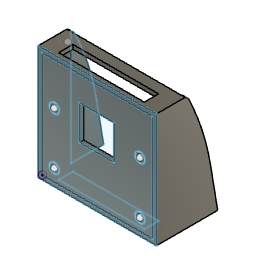
Drone_PiCameraCase v4 (Autodesk Fusion 360 design; units mm, degrees)
Autodesk Fusion 360 part; units mm, degrees
sketch "Sketch2" plane through (0, 0, 0) normal (0, 1, 0) x (1, 0, 0)
  circle A0 centre (2.9671, -2.9729) radius 1.2
  circle A1 centre (23.9671, -2.9729) radius 1.2
  circle A2 centre (23.9671, -15.7229) radius 1.2
  circle A3 centre (2.9671, -15.7229) radius 1.2
  line L0 (9.1497, -11.5214) -> (9.1497, -19.9214)
  line L1 (9.1497, -19.9214) -> (17.5497, -19.9214)
  line L2 (17.5497, -19.9214) -> (17.5497, -11.5214)
  line L3 (17.5497, -11.5214) -> (9.1497, -11.5214)
  line L4 (26.9671, 0.0271) -> (26.9671, -25.9729)
  line L5 (26.9671, -25.9729) -> (-0.0329, -25.9729)
  line L6 (-0.0329, -25.9729) -> (-0.0329, 0.0271)
  line L7 (-0.0329, 0.0271) -> (26.9671, 0.0271)
  line L8 (-1, -27) -> (28, -27)
  line L9 (28, -27) -> (28, 1)
  line L10 (28, 1) -> (-1, 1)
  line L11 (-1, 1) -> (-1, -27)
  dimension "d3" = 2.4
  dimension "d4" = 2.4
  dimension "d5" = 2.4
  dimension "d6" = 2.4
  dimension "d7" = 8.4
  dimension "d8" = 8.4
  constraint horizontal L8
  constraint vertical L9
  constraint horizontal L10
  constraint vertical L11
  measures "d3" diameter of A0
  measures "d4" diameter of A1
  measures "d5" diameter of A2
  measures "d6" diameter of A3
  measures "d7" distance of L0.start L0.end
  measures "d8" distance of L0.start L2.end
extrude "Extrude12" add sketch "Sketch2" along normal blind 1 contours L4 L5 L6 L7 makes body 1
extrude "Extrude11" add sketch "Sketch2" along normal blind 7 separate body contours L8 L9 L10 L11 makes body 2
extrude "Extrude13" add sketch "Sketch2" along normal blind 5 contours A0 | A1 | A2 | A3 bodies 1
sketch "Sketch5" plane through (0, 0, 0) normal (0, 0, 1) x (1, 0, 0)
  line L0 (3, 4.5) -> (24, 4.5)
  line L1 (24, 4.5) -> (24, 1)
  line L2 (24, 1) -> (3, 1)
  line L3 (3, 1) -> (3, 4.5)
  dimension "d37" = 21
  dimension "d38" = 3.5
  constraint horizontal L0
  constraint vertical L1
  constraint horizontal L2
  constraint vertical L3
  measures "d37" distance of L0.start L0.end
  measures "d38" distance of L0.start L2.end
extrude "Extrude14" cut sketch "Sketch5" along normal blind 30 bodies 1 2
extrude "Extrude15" add 4 faces at (2.555, 5, 16.0039) (23.555, 5, 16.0039) (23.0762, 5, 2.6783) (2.597, 5, 2.5741) along direction (0, -1, 0) blind 4 on bodies 1 bodies 1
sketch "Sketch6" plane through (0, 0, 0) normal (1, 0, 0) x (0, 1, 0)
  line L0 (7, -1) -> (15, -1)
  line L1 (15, -1) -> (13.2758, 9.3453)
  line L2 (8.8483, 24.0914) -> (8, 26)
  arc A0 (8, 26) -> (7, 27) centre (6.2, 25.2) ccw
  line L3 (7, 27) -> (7, -1)
  arc A1 (13.2758, 9.3453) -> (8.8483, 24.0914) centre (-46.8942, -0.683) ccw
  dimension "d43" = 61
  constraint horizontal L0
  constraint tangent L2 A0
  constraint perpendicular L0 L3
  constraint tangent L1 A1
  constraint tangent L2 A1
  measures "d43" radius of A1
extrude "Extrude16" add sketch "Sketch6" along normal blind 28 bodies 2
extrude "Extrude17" cut 1 faces at (0, 11.7586, 2.7728) along direction (1, 0, 0) blind 27 on bodies 2 bodies 2
extrude "Extrude18" add sketch "Sketch6" against normal blind 1 bodies 2
extrude "Extrude9" [suppressed]
